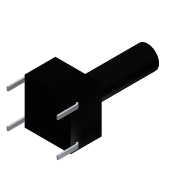
# Autodesk Inventor part: button
Saved by Autodesk Inventor 2015 SP1 (Build 190203100, 203)
## iProperties
Created: 2015-12-01
Part Number: button
Material: Generic
Document SubType Name: Modeling
Designer: User
Density: 1 g/cm^3
Appearance: Default
Mass: 0.208774 g
Surface Area: 2.69022 cm^2
Volume: 0.208774 cm^3
Author: User
Autodesk Inventor part; units mm, degrees
ref_plane "YZ Plane" through (0, 0, 0) normal (1, 0, 0) x (0, 1, 0)
ref_plane "XZ Plane" through (0, 0, 0) normal (0, 1, 0) x (-1, 0, 0)
sketch "Эскиз1" plane through (0, 0, 0) normal (0, 1, 0) x (-1, 0, 0)
  line L0 (3, -3) -> (-3, -3)
  line L1 (-3, -3) -> (-3, 3)
  line L2 (-3, 3) -> (3, 3)
  line L3 (3, 3) -> (3, -3)
  line L4 (4.2, 0) -> (-4.2, 0) projected
  line L5 (0, -4.2) -> (0, 4.2) projected
  point P0 (0, 0)
  dimension "d0" = 6
  dimension "d1" = 6
  constraints: 8 end point, 2 parallel, 1 horizontal, 1 perpendicular, 2 other
  measures "d0" distance of L0.end L1.end
  measures "d1" distance of L0.start L0.end
extrude "Выдавливание1" add sketch "Эскиз1" along normal blind 4
sketch "Эскиз2" plane through (0, 4, 0) normal (0, 1, 0) x (1, 0, 0)
  circle A0 centre (0, 0) radius 1.5
  dimension "d4" = 3
  constraints: 1 centre point, 1 coincident
  measures "d4" diameter of A0
ref_plane "РабПлоскость1" through (0, 13, 0) normal (0, 1, 0) x (1, 0, 0)
sketch "Эскиз3" plane through (0, 13, 0) normal (0, 1, 0) x (1, 0, 0)
  circle A0 centre (0, 0) radius 1.5
  dimension "d6" = 3
  constraints: 1 centre point, 1 coincident
  measures "d6" diameter of A0
loft "Лофт1" add profiles "Эскиз3", "Эскиз2"
sketch "Эскиз4" plane through (0, 0, 0) normal (0, 0, 1) x (1, 0, 0)
  line L0 (3, 0) -> (-3, 0) projected
  line L1 (3, 0) -> (3, 4) projected
  line L2 (-3, 4) -> (3, 4) projected
  line L3 (-3, 0) -> (-3, 4) projected
  arc A0 (3.25, 0.5) -> (3, 0.75) centre (3, 0.5) ccw
  line L4 (3.25, 0.5) -> (3.25, -2)
  line L5 (0, -5) -> (0, 16) projected
  arc A1 (-3, 0.75) -> (-3.25, 0.5) centre (-3, 0.5) ccw
  line L6 (-3.25, 0.5) -> (-3.25, -2)
  point P0 (0, 0)
  dimension "d11" = 0.5
  dimension "d12" = 0.5
  dimension "d13" = 2
  constraints: 4 end point, 4 point on circle, 4 symmetric about line, 2 centre point, 2 point on line, 1 vertical, 1 other
  measures "d11" diameter of A0
  measures "d12" distance from line of L0 A0.centre
  measures "d13" distance from line of L0 L4.end
sketch "Эскиз5" plane through (3, 0, 3) normal (1, 0, 0) x (0, 0, -1)
  line L0 (3.7546, 0.75) -> (2.4212, 0.75)
  line L1 (0.5, 0.85) -> (1, 0.85)
  line L2 (1, 0.85) -> (1, 0.65)
  line L3 (1, 0.65) -> (0.5, 0.65)
  line L4 (0.5, 0.65) -> (0.5, 0.85)
  line L5 (3, -5) -> (3, 16) projected
  line L6 (5.5, 0.85) -> (5, 0.85)
  line L7 (5, 0.85) -> (5, 0.65)
  line L8 (5, 0.65) -> (5.5, 0.65)
  line L9 (5.5, 0.65) -> (5.5, 0.85)
  line L10 (3, 0.75) -> (3, 0.5) projected
  point P0 (3, 0)
  dimension "d14" = 0.5
  dimension "d15" = 0.2
  dimension "d16" = 2
  constraints: 18 end point, 4 symmetric about line, 2 horizontal, 2 parallel, 1 perpendicular, 1 point on line, 1 other
  measures "d14" distance of L2.end L3.end
  measures "d15" distance of L1.end L2.end
  measures "d16" distance between parallel lines of L5 L2
sketch "Эскиз6" plane through (-3, 0, -3) normal (-1, 0, 0) x (0, 0, 1)
  line L0 (5.5, 0.85) -> (5, 0.85) projected
  line L1 (5.5, 0.65) -> (5.5, 0.85) projected
  line L2 (5, 0.65) -> (5.5, 0.65) projected
  line L3 (5, 0.85) -> (5, 0.65) projected
  line L4 (0, 0) -> (6, 0) projected
  line L5 (0, 0) -> (0, 4) projected
  line L6 (6, 4) -> (0, 4) projected
  line L7 (6, 0) -> (6, 4) projected
  line L8 (0.5, 0.85) -> (1, 0.85) projected
  line L9 (1, 0.85) -> (1, 0.65) projected
  line L10 (1, 0.65) -> (0.5, 0.65) projected
  line L11 (0.5, 0.65) -> (0.5, 0.85) projected
  point P0 (3, 0)
sweep "Сдвиг1" add profiles "Эскиз5" path "Эскиз4" path curves A0 L4
sweep "Сдвиг2" add profiles "Эскиз6" path "Эскиз4" path curves A1 L6 contours L1 L2 L3 L0 | L8 L9 L10 L11
sketch "Эскиз7" plane through (0, 0, 0) normal (0, -1, 0) x (1, 0, 0)
  line L0 (-3.35, -2) -> (-3.35, -2.5) projected
  line L1 (-3.35, -2.5) -> (-3.15, -2.5) projected
  line L2 (-3.15, -2.5) -> (-3.15, -2) projected
  line L3 (-3.15, -2) -> (-3.35, -2) projected
  circle A0 centre (-3.25, -2.25) radius 0.2693
  point P0 (0, 0)
  constraints: 3 point on circle, 1 centre point
equation "\"d1\" = d0"
